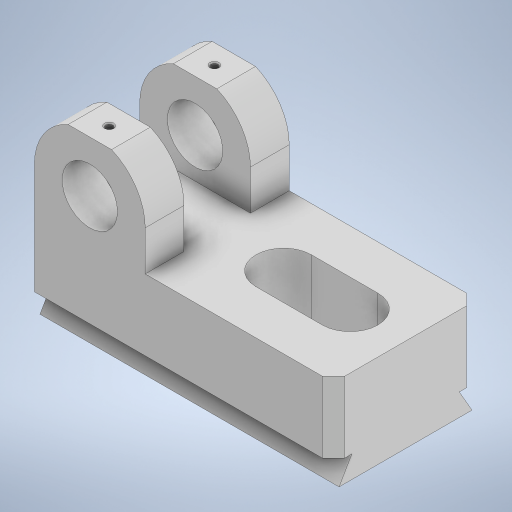
# Autodesk Inventor part: Schwalbenschwanzhalterung
Saved by Autodesk Inventor 2024 (Build 280153000, 153)
## iProperties
Created: 2023-09-21
Part Number: Schwalbenschwanzhalterung
Material: Generisch
Document SubType Name: Modeling
Designer: DEBIESTAI
Density: 1 g/cm^3
Appearance: Vorgabe
Author: DEBIESTAI
Autodesk Inventor part; units mm, degrees
ref_plane "YZ Plane" through (0, 0, 0) normal (1, 0, 0) x (0, 1, 0)
ref_plane "XZ Plane" through (0, 0, 0) normal (0, 1, 0) x (-1, 0, 0)
ref_plane "XY Plane" through (0, 0, 0) normal (0, 0, 1) x (1, 0, 0)
sketch "Skizze1" plane through (0, 0, 0) normal (1, 0, 0) x (0, 1, 0)
  line L0 (-30, -26) -> (30, -26)
  line L1 (30, -26) -> (24.2265, -16)
  line L2 (24.2265, -16) -> (32.5, -16)
  line L3 (32.5, -16) -> (32.5, 16)
  line L4 (32.5, 16) -> (-32.5, 16)
  line L5 (-32.5, 16) -> (-32.5, -16)
  line L6 (-32.5, -16) -> (-24.2265, -16)
  line L7 (-24.2265, -16) -> (-30, -26)
  point P0 (0, 0)
  dimension "d0" = 60
  dimension "d1" = 65
  dimension "d2" = 2.5
  dimension "d3" = 10
  dimension "d4" = 42
  dimension "d5" = 60
  dimension "d6" = 60
  dimension "d7" = 16
  dimension "d8" = 32.5
  constraints: 16 end point, 3 perpendicular, 2 point on line, 1 horizontal, 1 parallel
  measures "d0" distance of L0.start L0.end
  measures "d1" distance of L3.end L4.end
  measures "d2" distance from line of L0.start L5
  measures "d3" distance between parallel lines of L0 L2
  measures "d4" distance between parallel lines of L0 L4
  measures "d5" angle of L2 L1
  measures "d6" angle of L6 L7
  measures "d7" distance from line of L4 point (0, 0)
  measures "d8" distance from line of L3 point (0, 0)
extrude "Extrusion1" add sketch "Skizze1" against normal blind 135
sketch "Skizze2" plane through (0, -32.5, 16) normal (0, 0, 1) x (1, 0, 0)
  line L0 (0, 0) -> (-135, 0) projected
  line L1 (-135, 0) -> (-85, 0)
  line L2 (-85, 0) -> (-85, 17.5)
  line L3 (-85, 17.5) -> (-135, 17.5)
  line L4 (-135, 17.5) -> (-135, 0)
  line L5 (-135, 65) -> (-135, 56.7265) projected
  line L6 (-135, 65) -> (-85, 65)
  line L7 (-85, 65) -> (-85, 47.5)
  line L8 (-85, 47.5) -> (-135, 47.5)
  line L9 (-135, 47.5) -> (-135, 65)
  point P0 (0, 32.5)
  point P1 (-85, 0)
  dimension "d11" = 50
  dimension "d12" = 17.5
  dimension "d13" = 50
  dimension "d14" = 17.5
  constraints: 16 end point, 4 parallel, 2 horizontal, 2 perpendicular
  measures "d11" distance of L2.end L3.end
  measures "d12" distance of L3.end L0.end
  measures "d13" distance of L7.end L8.end
  measures "d14" distance of L6.end L7.end
extrude "Extrusion2" add sketch "Skizze2" along normal blind 43
fillet "Rundung1" radius 25 4 edges at (-85, -23.75, 59) (-135, -23.75, 59) (-85, 23.75, 59) (-135, 23.75, 59)
sketch "Skizze3" plane through (0, -32.5, -16) normal (0, -1, 0) x (1, 0, 0)
  line L0 (-85, 32) -> (-85, 50) projected
  line L1 (0, -10) -> (-135, -10) projected
  point P0 (0, 16)
  point P1 (-110, 50)
  dimension "d25" = 25
  dimension "d26" = 60
  measures "d25" distance from line of L0 point (-110, 50)
  measures "d26" distance from line of L1 point (-110, 50)
hole "Bohrung1" at (-110, -32.5, 34) direction (0, 1, 0) diameter 25 end through all
sketch "Skizze4" plane through (0, -32.5, 16) normal (0, 0, 1) x (1, 0, 0)
  line L0 (-55, 32.5) -> (-25, 32.5) construction
  line L1 (-55, 20) -> (-25, 20)
  line L2 (-25, 45) -> (-55, 45)
  arc A0 (-55, 45) -> (-55, 20) centre (-55, 32.5) ccw
  arc A1 (-25, 20) -> (-25, 45) centre (-25, 32.5) ccw
  line L3 (0, 65) -> (0, 0) projected
  line L4 (0, 0) -> (-85, 0) projected
  point P0 (0, 32.5)
  point P1 (-40, 32.5)
  dimension "d27" = 30
  dimension "d28" = 25
  dimension "d29" = 32.5
  dimension "d30" = 25
  constraints: 8 end point, 4 point on circle, 4 tangent, 2 centre point, 1 horizontal, 1 midpoint, 1 parallel
  measures "d27" distance of L0.start L0.end
  measures "d28" distance from line of L3 L0.end
  measures "d29" distance between parallel lines of L4 L0
  measures "d30" distance between parallel lines of L1 L2
extrude "Extrusion3" cut sketch "Skizze4" against normal through all
sketch "Skizze5" plane through (0, -32.5, -16) normal (0, -1, 0) x (1, 0, 0)
  line L0 (-135, 77) -> (-85, 77)
  line L1 (-85, 77) -> (-85, 73)
  line L2 (-85, 73) -> (-135, 73)
  line L3 (-135, 73) -> (-135, 77)
  line L4 (-85, 32) -> (-85, 50) projected
  line L5 (-135, 0) -> (-135, 50) projected
  arc A0 (-85, 50) -> (-135, 50) centre (-110, 50) ccw projected
  point P0 (0, 16)
  point P1 (-110, 73)
  point P2 (-110, 75)
  dimension "d33" = 2
  dimension "d34" = 4
  constraints: 8 end point, 2 collinear, 2 parallel, 1 horizontal, 1 midpoint, 1 perpendicular, 1 point on circle
  measures "d33" distance of point (-110, 73) point (-110, 75)
  measures "d34" distance of L2.end L0.start
extrude "Extrusion4" cut sketch "Skizze5" against normal through all
sketch "Skizze6" plane through (-119.798, -32.5, 57) normal (0, 0, 1) x (1, 0, 0)
  line L0 (119.798, 65) -> (119.798, 0) projected
  line L1 (0, 65) -> (19.5959, 65) projected
  point P0 (119.798, 32.5)
  point P1 (9.798, 8.75)
  point P2 (9.798, 56.25)
  dimension "d44" = 110
  dimension "d45" = 110
  dimension "d46" = 47.5
  dimension "d47" = 8.75
  measures "d44" distance from line of L0 point (9.798, 56.25)
  measures "d45" distance from line of L0 point (9.798, 8.75)
  measures "d46" distance of point (9.798, 8.75) point (9.798, 56.25)
  measures "d47" distance from line of L1 point (9.798, 56.25)
hole "Bohrung2" at (-110, -23.75, 57) at (-110, 23.75, 57) direction (0, 0, -1) diameter 3.242 depth 14 thread size "M4x0.7" class "6H" standard "ISO Metric profile"
chamfer "Fasen1" distance 0.5 angle 45 2 edges at (-110, 25.371, 57) (-110, -22.129, 57)
chamfer "Fasen2" distance 5 angle 45 2 edges at (0, -32.5, 0) (0, 32.5, 0)
